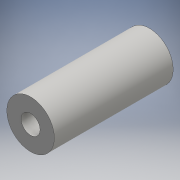
# Autodesk Inventor part: 机械爪六角筒
Saved by Autodesk Inventor 2016 (Build 200138000, 138)
## iProperties
Created: 2019-05-18
Part Number: 机械爪六角筒
Material: 常规
Document SubType Name: Modeling
Designer: oldboy
Density: 1 g/cm^3
Appearance: 默认
Author: oldboy
Autodesk Inventor part; units mm, degrees
ref_plane "YZ Plane" through (0, 0, 0) normal (1, 0, 0) x (0, 1, 0)
ref_plane "XZ Plane" through (0, 0, 0) normal (0, 1, 0) x (-1, 0, 0)
ref_plane "XY Plane" through (0, 0, 0) normal (0, 0, 1) x (1, 0, 0)
sketch "草图1" plane through (0, 0, 0) normal (0, 1, 0) x (-1, 0, 0)
  circle A0 centre (0, 0) radius 5
  line L0 (2.95, -1.7032) -> (0, -3.4064)
  line L1 (0, -3.4064) -> (-2.95, -1.7032)
  line L2 (-2.95, -1.7032) -> (-2.95, 1.7032)
  line L3 (-2.95, 1.7032) -> (0, 3.4064)
  line L4 (0, 3.4064) -> (2.95, 1.7032)
  line L5 (2.95, 1.7032) -> (2.95, -1.7032)
  point P0 (2.95, 0)
  dimension "d0" = 10
  constraints: 12 end point, 1 centre point, 1 coincident, 1 midpoint, 13 other
  measures "d0" diameter of A0
extrude "拉伸1" add sketch "草图1" along normal blind 25
sketch "草图3" plane through (0, 0, 0) normal (0, -1, 0) x (1, 0, 0)
  circle A0 centre (0, 0) radius 2
  circle A1 centre (0, 0) radius 5 projected
  dimension "d7" = 4
  constraints: 1 centre point, 1 coincident
  measures "d7" diameter of A0
extrude "拉伸3" add sketch "草图3" against normal blind 3
